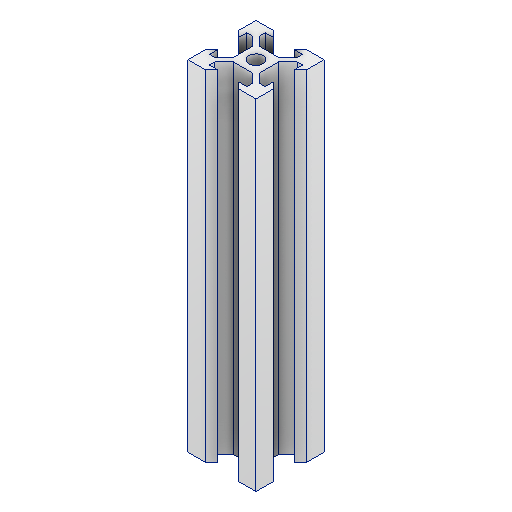
# Autodesk Inventor part: vslot_100mm
Saved by Autodesk Inventor 2023 (Build 270158000, 158)
## iProperties
Created: 2023-12-19
Part Number: vslot_100mm
Material: Aluminum 6061
Document SubType Name: Modeling
Designer: diego
Density: 2.7 g/cm^3
Appearance: Aluminum - Flat
Mass: 45.2751 g
Surface Area: 162.835 cm^2
Volume: 16.7686 cm^3
Author: diego
Autodesk Inventor part; units mm, degrees
ref_plane "YZ Plane" through (0, 0, 0) normal (1, 0, 0) x (0, 1, 0)
ref_plane "XZ Plane" through (0, 0, 0) normal (0, 1, 0) x (-1, 0, 0)
ref_plane "XY Plane" through (0, 0, 0) normal (0, 0, 1) x (1, 0, 0)
sketch "Sketch1" plane through (0, 0, 0) normal (0, 1, 0) x (-1, 0, 0)
  circle A0 centre (0, 0) radius 2.1
  line L0 (0, -3.9007) -> (-2.84, -3.9007)
  line L1 (-5.4993, -8.2) -> (-3.1, -8.2)
  line L2 (-3.1, -8.2) -> (-4.9, -10)
  line L3 (-4.9, -10) -> (-10, -10)
  line L4 (-10, -10) -> (-10, -4.9)
  line L5 (-10, -4.9) -> (-8.2, -3.1)
  line L6 (-8.2, -3.1) -> (-8.2, -5.4993)
  line L7 (-3.9007, -2.84) -> (-3.9007, 0)
  line L8 (-3.9007, 0) -> (-2.1, 0)
  line L9 (0, -3.9007) -> (0, -2.1) construction
  line L10 (-5.4993, -8.2) -> (-5.4993, -6.56)
  line L11 (-5.4993, -6.56) -> (-2.84, -3.9007)
  line L12 (-3.9007, -2.84) -> (-6.56, -5.4993)
  line L13 (-6.56, -5.4993) -> (-8.2, -5.4993)
  line L14 (6.56, -5.4993) -> (3.9007, -2.84)
  line L15 (3.1, -8.2) -> (5.4993, -8.2)
  line L16 (5.4993, -6.56) -> (5.4993, -8.2)
  line L17 (8.2, -5.4993) -> (8.2, -3.1)
  line L18 (8.2, -5.4993) -> (6.56, -5.4993)
  line L19 (8.2, -3.1) -> (10, -4.9)
  line L20 (4.9, -10) -> (3.1, -8.2)
  line L21 (10, -4.9) -> (10, -10)
  line L22 (10, -10) -> (4.9, -10)
  line L23 (2.84, -3.9007) -> (0, -3.9007)
  line L24 (0, -3.9007) -> (0, -2.1) construction
  line L25 (3.9007, 0) -> (2.1, 0)
  line L26 (3.9007, 0) -> (3.9007, -2.84)
  line L27 (2.84, -3.9007) -> (5.4993, -6.56)
  line L28 (5.4993, 6.56) -> (2.84, 3.9007)
  line L29 (8.2, 3.1) -> (8.2, 5.4993)
  line L30 (6.56, 5.4993) -> (8.2, 5.4993)
  line L31 (5.4993, 8.2) -> (3.1, 8.2)
  line L32 (5.4993, 8.2) -> (5.4993, 6.56)
  line L33 (3.1, 8.2) -> (4.9, 10)
  line L34 (10, 4.9) -> (8.2, 3.1)
  line L35 (4.9, 10) -> (10, 10)
  line L36 (10, 10) -> (10, 4.9)
  line L37 (3.9007, 2.84) -> (3.9007, 0)
  line L38 (3.9007, 0) -> (2.1, 0) construction
  line L39 (0, 3.9007) -> (0, 2.1)
  line L40 (0, 3.9007) -> (2.84, 3.9007)
  line L41 (3.9007, 2.84) -> (6.56, 5.4993)
  line L42 (-6.56, 5.4993) -> (-3.9007, 2.84)
  line L43 (-3.1, 8.2) -> (-5.4993, 8.2)
  line L44 (-5.4993, 6.56) -> (-5.4993, 8.2)
  line L45 (-8.2, 5.4993) -> (-8.2, 3.1)
  line L46 (-8.2, 5.4993) -> (-6.56, 5.4993)
  line L47 (-8.2, 3.1) -> (-10, 4.9)
  line L48 (-4.9, 10) -> (-3.1, 8.2)
  line L49 (-10, 4.9) -> (-10, 10)
  line L50 (-10, 10) -> (-4.9, 10)
  line L51 (-2.84, 3.9007) -> (0, 3.9007)
  line L52 (0, 3.9007) -> (0, 2.1) construction
  line L53 (-3.9007, 0) -> (-2.1, 0) construction
  line L54 (-3.9007, 0) -> (-3.9007, 2.84)
  line L55 (-2.84, 3.9007) -> (-5.4993, 6.56)
  point P0 (0, -3.0003)
  point P1 (-3.0003, 0)
  point P2 (0, -3.0003)
  point P3 (3.0003, 0)
  point P4 (3.0003, 0)
  point P5 (0, 3.0003)
  point P6 (0, 3.0003)
  point P7 (-3.0003, 0)
  dimension "d0" = 4.2
  dimension "d2" = 45
  dimension "d3" = 3.1
  dimension "d4" = 2.84
  dimension "d7" = 10
  dimension "d8" = 10
  dimension "d9" = 1.5
  dimension "d10" = 1.8
  dimension "d11" = 1.64
  dimension "d14" = 360
  constraints: 112 end point, 6 equal length, 6 parallel, 4 perpendicular, 2 midpoint, 2 point on circle, 1 centre point, 1 coincident, 1 horizontal, 1 horizontal alignment, 1 vertical, 1 vertical alignment, 129 other
  measures "d0" diameter of A0
  measures "d2" angle of L9 L2
  measures "d3" distance from line of L8 L5.end
  measures "d4" distance of L7.end L7.start
  measures "d7" distance between parallel lines of L8 L3
  measures "d8" distance from line of point (0, 0) L4
  measures "d9" distance between parallel lines of L11 L12
  measures "d10" distance between parallel lines of L3 L1
  measures "d11" distance of L12.end L6.end
extrude "Extrusion1" add sketch "Sketch1" along normal mid plane 100 contours L25 L26 L14 L18 L17 L19 L21 L22 L20 L15 L16 L27 L23 L0 L11 L10 L1 L2 L3 L4 L5 L6 L13 L12 L7 L8 A0 | A0 L39 L40 L28 L32 L31 L33 L35 L36 L34 L29 L30 L41 L37 L25 | A0 L8 L54 L42 L46 L45 L47 L49 L50 L48 L43 L44 L55 L51 L39
body "Solid1"
